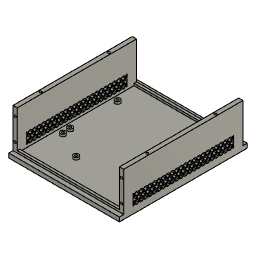
Base v16 (Autodesk Fusion 360 design; units mm, degrees)
Autodesk Fusion 360 part; units mm, degrees
sketch "Sketch1" plane through (0, 0, 0) normal (0, 0, 1) x (1, 0, 0)
  line L0 (0, 0) -> (130, 0)
  line L1 (130, 0) -> (130, 150)
  line L2 (130, 150) -> (0, 150)
  line L3 (0, 150) -> (0, 0)
  dimension "d1" = 130
  dimension "d2" = 150
  constraint horizontal L0
  constraint vertical L1
  constraint horizontal L2
  constraint vertical L3
  constraint coincident L0.start L3.end
  measures "d1" distance of L0.start L0.end
  measures "d2" distance of L0.start L2.end
extrude "Extrude1" add sketch "Sketch1" along normal blind 5 makes body 1
sketch "Sketch2" plane through (0, 0, 5) normal (0, 0, 1) x (-1, 0, 0)
  line L0 (0, -150) -> (0, 0)
  line L1 (0, 0) -> (-130, 0)
  line L2 (-130, 0) -> (-130, -150)
  line L3 (-130, -150) -> (0, -150)
  line L4 (0, -45) -> (-130, -45) construction
  line L5 (-5, 0) -> (-5, -150) construction
  line L6 (-125, 0) -> (-125, -150) construction
  line L7 (-7.569, -120.53) -> (-122.431, -120.53) construction
  line L8 (-122.431, -120.53) -> (-122.431, -55) construction
  line L9 (-122.431, -55) -> (-7.569, -55) construction
  line L10 (-7.569, -55) -> (-7.569, -120.53) construction
  line L11 (-12.2, -115.615) -> (-117.8, -115.615) construction
  line L12 (-117.8, -115.615) -> (-117.8, -59.915) construction
  line L13 (-117.8, -59.915) -> (-12.2, -59.915) construction
  line L14 (-12.2, -59.915) -> (-12.2, -115.615) construction
  circle A0 centre (-12.2, -115.615) radius 3
  circle A1 centre (-117.8, -115.615) radius 3
  circle A2 centre (-12.2, -59.915) radius 3
  circle A3 centre (-117.8, -59.915) radius 3
  line L15 (-7.6129, -53) -> (-50.1129, -53) construction
  line L16 (-50.1129, -53) -> (-50.1129, -32) construction
  line L17 (-50.1129, -32) -> (-7.6129, -32) construction
  line L18 (-7.6129, -32) -> (-7.6129, -53) construction
  circle A4 centre (-13.1629, -50.46) radius 3
  circle A5 centre (-44.5629, -34.54) radius 3
  point P0 (-12.2, -115.615)
  point P1 (-117.8, -115.615)
  point P2 (-117.8, -59.915)
  point P3 (-12.2, -59.915)
  dimension "d5" = 45
  dimension "d6" = 5
  dimension "d7" = 5
  dimension "d8" = 114.862
  dimension "d9" = 65.53
  dimension "d10" = 2.569
  dimension "d11" = 10
  dimension "d12" = 105.6
  dimension "d13" = 55.7
  dimension "d14" = 4.631
  dimension "d15" = 4.915
  dimension "d16" = 6
  dimension "d17" = 6
  dimension "d18" = 6
  dimension "d19" = 6
  dimension "d25" = 42.5
  dimension "d26" = 21
  dimension "d27" = 6
  dimension "d28" = 6
  dimension "d29" = 5.55
  dimension "d30" = 2.54
  dimension "d31" = 5.55
  dimension "d32" = 2.54
  dimension "d33" = 2
  constraint coincident L0 L4.start
  constraint coincident L2 L4.end
  constraint perpendicular L2 L4
  constraint coincident L1 L5.start
  constraint coincident L3 L5.end
  constraint perpendicular L3 L5
  constraint coincident L1 L6.start
  constraint coincident L3 L6.end
  constraint perpendicular L3 L6
  constraint horizontal L7
  constraint vertical L8
  constraint horizontal L9
  constraint vertical L10
  constraint horizontal L11
  constraint vertical L12
  constraint horizontal L13
  constraint vertical L14
  constraint coincident P0 L11.start
  constraint coincident P1 L11.end
  constraint coincident P3 L13.end
  constraint coincident P2 L12.end
  constraint horizontal L15
  constraint vertical L16
  constraint horizontal L17
  constraint vertical L18
  measures "d5" distance of L1 L4
  measures "d6" distance of L0 L5
  measures "d7" distance of L2 L6
  measures "d8" distance of L7.start L7.end
  measures "d9" distance of L7.start L9.end
  measures "d10" distance of L5 L10
  measures "d11" distance of L4 L9
  measures "d12" distance of P0 P1
  measures "d13" distance of P0 P3
  measures "d14" distance of L8 L12
  measures "d15" distance of L7 L11
  measures "d16" diameter of A0
  measures "d17" diameter of A1
  measures "d18" diameter of A2
  measures "d19" diameter of A3
  measures "d25" distance of L15.start L15.end
  measures "d26" distance of L15.start L17.end
  measures "d27" diameter of A4
  measures "d28" diameter of A5
  measures "d29" distance of L18 A4.centre
  measures "d30" distance of L15 A4.centre
  measures "d31" distance of L16 A5.centre
  measures "d32" distance of L17 A5.centre
  measures "d33" distance of L9 L15
extrude "Extrude2" add sketch "Sketch2" along normal blind 3 contours A0 | A1 | A2 | A3 | A4 | A5 bodies 1
sketch "Sketch5" plane through (0, 0, 8) normal (0, 0, 1) x (-1, 0, 0)
  circle A0 centre (-12.2, -115.615) radius 3
  point P0 (-12.2, -115.615)
  constraint coincident P0 A0.centre
sketch "Sketch6" plane through (0, 0, 8) normal (0, 0, 1) x (-1, 0, 0)
  circle A0 centre (-117.8, -115.615) radius 3
  point P0 (-117.8, -115.615)
  constraint coincident P0 A0.centre
sketch "Sketch7" plane through (0, 0, 8) normal (0, 0, 1) x (-1, 0, 0)
  circle A0 centre (-12.2, -59.915) radius 3
  point P0 (-12.2, -59.915)
  constraint coincident P0 A0.centre
sketch "Sketch8" plane through (0, 0, 8) normal (0, 0, 1) x (-1, 0, 0)
  circle A0 centre (-117.8, -59.915) radius 3
  point P0 (-117.8, -59.915)
  constraint coincident P0 A0.centre
sketch "Sketch9" plane through (0, 0, 8) normal (0, 0, 1) x (-1, 0, 0)
  circle A0 centre (-13.1629, -50.46) radius 3
  point P0 (-13.1629, -50.46)
  constraint coincident P0 A0.centre
sketch "Sketch10" plane through (0, 0, 8) normal (0, 0, 1) x (-1, 0, 0)
  circle A0 centre (-44.5629, -34.54) radius 3
  point P0 (-44.5629, -34.54)
  constraint coincident P0 A0.centre
hole "Hole1" at (117.8, 115.615, 8) at (12.2, 115.615, 8) at (12.2, 59.915, 8) at (117.8, 59.915, 8) at (44.5629, 34.54, 8) at (13.1629, 50.46, 8) direction (0, 0, -1) diameter 2.65 depth 7.5 tip angle 180 bodies 1
sketch "Sketch11" plane through (0, 0, 5) normal (0, 0, 1) x (-1, 0, 0)
  circle A0 centre (-44.5629, -34.54) radius 3
  circle A1 centre (-117.8, -115.615) radius 3
  circle A2 centre (-117.8, -59.915) radius 3
  circle A3 centre (-13.1629, -50.46) radius 3
  circle A4 centre (-12.2, -115.615) radius 3
  circle A5 centre (-12.2, -59.915) radius 3
  line L0 (0, -150) -> (0, 0)
  line L1 (0, 0) -> (-130, 0)
  line L2 (-130, 0) -> (-130, -150)
  line L3 (-130, -150) -> (0, -150)
  line L4 (0, -145) -> (-130, -145) construction
  line L5 (0, -5) -> (-130, -5) construction
  line L6 (0, -145) -> (-5, -145)
  line L7 (-5, -145) -> (-5, -5)
  line L8 (-5, -5) -> (0, -5)
  line L9 (0, -5) -> (0, -145)
  line L10 (-130, -145) -> (-125, -145)
  line L11 (-125, -145) -> (-125, -5)
  line L12 (-125, -5) -> (-130, -5)
  line L13 (-130, -5) -> (-130, -145)
  dimension "d34" = 5
  dimension "d35" = 5
  dimension "d36" = 5
  dimension "d37" = 5
  constraint coincident L0 L4.start
  constraint coincident L2 L4.end
  constraint perpendicular L2 L4
  constraint coincident L0 L5.start
  constraint coincident L2 L5.end
  constraint perpendicular L2 L5
  constraint horizontal L6
  constraint vertical L7
  constraint horizontal L8
  constraint vertical L9
  constraint coincident L5 L7.end
  constraint horizontal L10
  constraint vertical L11
  constraint horizontal L12
  constraint vertical L13
  constraint coincident L5 L11.end
  measures "d34" distance of L3 L4
  measures "d35" distance of L1 L5
  measures "d36" distance of L7 L9
  measures "d37" distance of L11 L13
extrude "Extrude3" add sketch "Sketch11" along normal blind 46 contours L0 L6 L7 L8 L9 | L2 L10 L11 L12 L13 bodies 1
sketch "Sketch12" plane through (0, 5, 0) normal (0, -1, 0) x (1, 0, 0)
  line L0 (0, 5) -> (5, 5)
  line L1 (5, 5) -> (5, 51)
  line L2 (5, 51) -> (0, 51)
  line L3 (0, 51) -> (0, 5)
  point P0 (2.5, 41)
  point P1 (2.5, 15)
  dimension "d40" = 10
  dimension "d41" = 10
  measures "d40" distance of L2 P0
  measures "d41" distance of L0 P1
sketch "Sketch13" plane through (0, 5, 0) normal (0, -1, 0) x (1, 0, 0)
  line L0 (125, 5) -> (130, 5)
  line L1 (130, 5) -> (130, 51)
  line L2 (130, 51) -> (125, 51)
  line L3 (125, 51) -> (125, 5)
  point P0 (127.5, 41)
  point P1 (127.5, 15)
  dimension "d42" = 10
  dimension "d43" = 10
  measures "d42" distance of L2 P0
  measures "d43" distance of L0 P1
sketch "Sketch14" plane through (0, 145, 0) normal (0, 1, 0) x (-1, 0, 0)
  line L0 (-130, 5) -> (-125, 5)
  line L1 (-125, 5) -> (-125, 51)
  line L2 (-125, 51) -> (-130, 51)
  line L3 (-130, 51) -> (-130, 5)
  point P0 (-127.5, 41)
  point P1 (-127.5, 15)
  dimension "d47" = 10
  dimension "d48" = 10
  measures "d47" distance of L2 P0
  measures "d48" distance of L0 P1
sketch "Sketch15" plane through (0, 145, 0) normal (0, 1, 0) x (-1, 0, 0)
  line L0 (-5, 5) -> (0, 5)
  line L1 (0, 5) -> (0, 51)
  line L2 (0, 51) -> (-5, 51)
  line L3 (-5, 51) -> (-5, 5)
  point P0 (-2.5, 41)
  point P1 (-2.5, 15)
  dimension "d49" = 10
  dimension "d50" = 10
  measures "d49" distance of L2 P0
  measures "d50" distance of L0 P1
hole "Hole3" at (2.5, 5, 41) at (2.5, 5, 15) at (127.5, 5, 15) at (127.5, 5, 41) direction (0, 1, 0) diameter 2.65 depth 10 tip angle 180 bodies 1
hole "Hole4" at (127.5, 145, 41) at (127.5, 145, 15) at (2.5, 145, 41) at (2.5, 145, 15) direction (0, -1, 0) diameter 2.65 depth 10 tip angle 180 bodies 1
sketch "Sketch16" plane through (0, 0, 5) normal (0, 0, 1) x (-1, 0, 0)
  line L0 (-125, -145) -> (-130, -145)
  line L1 (-130, -145) -> (-130, -150)
  line L2 (-130, -150) -> (0, -150)
  line L3 (0, -150) -> (0, -145)
  line L4 (0, -145) -> (-5, -145)
  line L5 (-5, -145) -> (-5, -5)
  line L6 (-5, -5) -> (0, -5)
  line L7 (0, -5) -> (0, 0)
  line L8 (0, 0) -> (-130, 0)
  line L9 (-130, 0) -> (-130, -5)
  line L10 (-130, -5) -> (-125, -5)
  line L11 (-125, -5) -> (-125, -145)
  circle A0 centre (-12.2, -59.915) radius 3
  circle A1 centre (-12.2, -115.615) radius 3
  circle A2 centre (-13.1629, -50.46) radius 3
  circle A3 centre (-117.8, -59.915) radius 3
  circle A4 centre (-117.8, -115.615) radius 3
  circle A5 centre (-44.5629, -34.54) radius 3
  line L12 (-5, -5) -> (-125, -5)
  line L13 (-125, -5) -> (-125, -8)
  line L14 (-125, -8) -> (-5, -8)
  line L15 (-5, -8) -> (-5, -5)
  line L16 (-5, -145) -> (-125, -145)
  line L17 (-125, -145) -> (-125, -142)
  line L18 (-125, -142) -> (-5, -142)
  line L19 (-5, -142) -> (-5, -145)
  dimension "d57" = 120
  dimension "d58" = 3
  dimension "d61" = 3
  constraint horizontal L12
  constraint vertical L13
  constraint horizontal L14
  constraint vertical L15
  constraint coincident L5.end L6.start
  constraint horizontal L16
  constraint vertical L17
  constraint horizontal L18
  constraint vertical L19
  constraint coincident L4.end L5.start
  measures "d57" distance of L5.end L10.end
  measures "d58" distance of L4.end L18.end
  measures "d61" distance of L12 L14
extrude "Extrude4" add sketch "Sketch16" along normal blind 2.5 contours L5 L11 L16 L17 L18 L19 | L5 L11 L12 L13 L14 L15 bodies 1
sketch "Sketch18" plane through (0, 0, 51) normal (0, 0, 1) x (-1, 0, 0)
  line L0 (0, -5) -> (-5, -5)
  line L1 (-5, -5) -> (-5, -145)
  line L2 (-5, -145) -> (0, -145)
  line L3 (0, -145) -> (0, -5)
  point P0 (-2.5, -115)
  point P1 (-2.5, -35)
  dimension "d62" = 30
  dimension "d63" = 30
  measures "d62" distance of L2 P0
  measures "d63" distance of L0 P1
sketch "Sketch19" plane through (0, 0, 51) normal (0, 0, 1) x (-1, 0, 0)
  line L0 (-130, -5) -> (-130, -145)
  line L1 (-130, -145) -> (-125, -145)
  line L2 (-125, -145) -> (-125, -5)
  line L3 (-125, -5) -> (-130, -5)
  point P0 (-127.5, -115)
  point P1 (-127.5, -35)
  dimension "d64" = 30
  dimension "d65" = 30
  measures "d64" distance of L3 P1
  measures "d65" distance of L1 P0
hole "Hole5" at (2.5, 115, 51) at (2.5, 35, 51) at (127.5, 35, 51) at (127.5, 115, 51) direction (0, 0, -1) diameter 2.65 depth 15 tip angle 180 bodies 1
sketch "Sketch20" plane through (0, 0, 0) normal (-1, 0, 0) x (0, -1, 0)
  line L0 (-150, 0) -> (0, 0)
  line L1 (0, 0) -> (0, 5)
  line L2 (0, 5) -> (-5, 5)
  line L3 (-5, 5) -> (-5, 51)
  line L4 (-5, 51) -> (-145, 51)
  line L5 (-145, 51) -> (-145, 5)
  line L6 (-145, 5) -> (-150, 5)
  line L7 (-150, 5) -> (-150, 0)
  line L8 (-145, 8) -> (-5, 8) construction
  line L9 (-134, 51) -> (-134, 8) construction
  line L10 (-16, 51) -> (-16, 8) construction
  line L11 (-5, 40) -> (-145, 40) construction
  line L12 (-134, 21) -> (-16, 21)
  line L13 (-16, 21) -> (-16, 8)
  line L14 (-16, 8) -> (-134, 8)
  line L15 (-134, 8) -> (-134, 21)
  line L16 (-134, 14.5) -> (-16, 14.5) construction
  line L17 (-75, 8) -> (-75, 21) construction
  line L18 (-77.6, 12.9989) -> (-75, 11.4978)
  line L19 (-75, 11.4978) -> (-72.4, 12.9989)
  line L20 (-72.4, 12.9989) -> (-72.4, 16.0011)
  line L21 (-72.4, 16.0011) -> (-75, 17.5022)
  line L22 (-75, 17.5022) -> (-77.6, 16.0011)
  line L23 (-77.6, 16.0011) -> (-77.6, 12.9989)
  line L24 (-72.4, 12.9989) -> (-69.8, 11.4978)
  line L25 (-69.8, 11.4978) -> (-67.2, 12.9989)
  line L26 (-67.2, 12.9989) -> (-67.2, 16.0011)
  line L27 (-67.2, 16.0011) -> (-69.8, 17.5022)
  line L28 (-69.8, 17.5022) -> (-72.4, 16.0011)
  line L29 (-72.4, 16.0011) -> (-72.4, 12.9989)
  line L30 (-75, 14.5) -> (-72.4, 14.5) construction
  line L31 (-75, 14.5) -> (-73.7, 16.7517) construction
  point P0 (-75, 14.5)
  point P1 (-69.8, 14.5)
  dimension "d69" = 8
  dimension "d70" = 11
  dimension "d71" = 11
  dimension "d72" = 11
  dimension "d75" = 118
  dimension "d76" = 13
  dimension "d78" = 5.2
  constraint coincident L5 L8.start
  constraint perpendicular L5 L8
  constraint coincident L4 L9.start
  constraint coincident L8 L9.end
  constraint perpendicular L8 L9
  constraint coincident L4 L10.start
  constraint coincident L8 L10.end
  constraint perpendicular L8 L10
  constraint coincident L3 L11.start
  constraint coincident L5 L11.end
  constraint perpendicular L5 L11
  constraint horizontal L12
  constraint vertical L13
  constraint horizontal L14
  constraint vertical L15
  constraint midpoint L8 L14
  constraint coincident L3 L8.end
  constraint midpoint L15 L16.start
  constraint midpoint L13 L16.end
  constraint midpoint L8 L17.start
  constraint midpoint L12 L17.end
  constraint midpoint L16 P0
  constraint vertical L23
  constraint coincident L20.end L21.start
  constraint coincident L19.end L20.start
  constraint coincident P0 L30.start
  constraint midpoint L20 L30.end
  constraint midpoint L21 L31.end
  measures "d69" distance of L0 L8
  measures "d70" distance of L5 L9
  measures "d71" distance of L3 L10
  measures "d72" distance of L4 L11
  measures "d75" distance of L13 L15
  measures "d76" distance of L12 L14
  measures "d78" distance of L20 L23
extrude "Extrude5" cut sketch "Sketch20" against normal up to surface (130 mm away) contours L12 L13 L14 L15 | L18 L19 L20 L21 L22 L23 L29 | L20 L24 L25 L26 L27 L28 L29 bodies 1
extrude "Extrude6" add sketch "Sketch20" against normal up to surface (130 mm away) thin wall 0.5 inside separate body contours L20 L24 L25 L26 L27 L28 L29 makes body 2
extrude "Extrude7" add sketch "Sketch20" against normal up to surface (130 mm away) thin wall 0.5 inside contours L18 L19 L20 L21 L22 L23 L29 bodies 2
pattern_linear "R-Pattern1" count 25 spacing 5.2 along (0, -1, 0) both ways count 5 spacing 5.2 along (0, -0.5, 0.866025) both ways of "Extrude7"
extrude "Extrude8" cut sketch "Sketch20" against normal up to surface (130 mm away) contours L12 L13 L14 L15 | L18 L19 L20 L21 L22 L23 L29 | L20 L24 L25 L26 L27 L28 L29 keep common part bodies 2
extrude "Extrude9" add sketch "Sketch20" against normal up to surface (130 mm away) thin wall 0.5 outside contours L12 L13 L14 L15 | L18 L19 L20 L21 L22 L23 L29 | L20 L24 L25 L26 L27 L28 L29 bodies 1 2
sketch "Sketch21" plane through (0, 15.5, 0) normal (0, -1, 0) x (1, 0, 0)
  line L0 (125, 7.5) -> (125, 21.5)
  line L1 (125, 21.5) -> (5, 21.5)
  line L2 (5, 21.5) -> (5, 7.5)
  line L3 (5, 7.5) -> (125, 7.5)
  line L4 (5, 21.5) -> (125, 21.5)
  line L5 (125, 21.5) -> (125, 7.5)
  line L6 (125, 7.5) -> (5, 7.5)
  line L7 (5, 7.5) -> (5, 21.5)
  constraint horizontal L4
  constraint vertical L5
  constraint horizontal L6
  constraint vertical L7
  constraint coincident L0.start L3.end
  constraint coincident L1.end L2.start
extrude "Extrude10" cut sketch "Sketch21" against normal up to surface (119 mm away) bodies 1
equation "Walls = 1 mm"
equation "Hexagon = 5.2 mm"
equation "d75 = Width - Walls * 2"
equation "d76 = Height - Walls * 2"
equation "d78 = Hexagon"
equation "Width = 120 mm"
equation "Height = 15 mm"
equation "d83 = Walls / 2"
equation "d86 = Walls / 2"
equation "d91 = Hexagon"
equation "d92 = Hexagon"
equation "d95 = Walls / 2"
